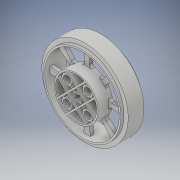
# Autodesk Inventor part: wheel
Saved by Autodesk Inventor 2019 (Build 230136000, 136)
## iProperties
Created: 2019-02-04
Part Number: wheel
Material: Generic
Document SubType Name: Modeling
Designer: david
Density: 1 g/cm^3
Appearance: Default
Author: david
Autodesk Inventor part; units mm, degrees
ref_plane "YZ Plane" through (0, 0, 0) normal (1, 0, 0) x (0, 1, 0)
ref_plane "XZ Plane" through (0, 0, 0) normal (0, 1, 0) x (-1, 0, 0)
ref_plane "XY Plane" through (0, 0, 0) normal (0, 0, 1) x (1, 0, 0)
sketch "Sketch1" plane through (0, 0, 0) normal (0, 0, 1) x (1, 0, 0)
  circle A0 centre (0, 0) radius 15
  dimension "d0" = 30
  constraints: 1 centre point, 1 coincident
  measures "d0" diameter of A0
extrude "Extrusion1" add sketch "Sketch1" along normal blind 10
ref_plane "Work Plane1" through (0, 0, -9) normal (0, 0, -1) x (-1, 0, 0)
sketch "Sketch2" plane through (0, 0, -9) normal (0, 0, -1) x (-1, 0, 0)
  circle A0 centre (0, 0) radius 26.65 construction
  circle A1 centre (0, 0) radius 29.5
  circle A2 centre (0, 0) radius 25.5
  dimension "d4" = 59
  dimension "d5" = 53.3
  dimension "d6" = 51
  constraints: 3 centre point, 3 coincident
  measures "d4" diameter of A1
  measures "d5" diameter of A0
  measures "d6" diameter of A2
extrude "Extrusion2" add sketch "Sketch2" against normal blind 15
sketch "Sketch3" plane through (0, 0, -9) normal (0, 0, -1) x (-1, 0, 0)
  circle A0 centre (0, 0) radius 29.5 projected
  circle A1 centre (0, 0) radius 26.75
  dimension "d9" = 53.5
  constraints: 1 centre point, 1 coincident
  measures "d9" diameter of A1
extrude "Extrusion3" cut sketch "Sketch3" against normal blind 2.1
sketch "Sketch4" plane through (0, 0, 6) normal (0, 0, 1) x (1, 0, 0)
  circle A0 centre (0, 0) radius 29.5 projected
  circle A1 centre (0, 0) radius 26.625
  dimension "d12" = 53.25
  constraints: 1 centre point, 1 coincident
  measures "d12" diameter of A1
extrude "Extrusion4" cut sketch "Sketch4" against normal blind 2.1
sketch "Sketch5" plane through (0, 0, 0) normal (0, 1, 0) x (-1, 0, 0)
  line L0 (15, 10) -> (-15, 10) projected
  line L1 (-25.5, 6) -> (25.5, 6) projected
  line L2 (-15, 0) -> (15, 0) projected
  line L3 (25.5, -9) -> (-25.5, -9) projected
  line L4 (-25.5, 6) -> (-25.5, -9)
  line L5 (-15, 0) -> (-25.5, 0)
  line L6 (-15, 0) -> (-15, 10)
  line L7 (-15, 2.5) -> (-25.5, 2.5)
  line L8 (0, 0) -> (0, 13.089) construction
  dimension "d19" = 2.5
  constraints: 10 end point, 3 point on line, 2 perpendicular, 2 vertical, 1 horizontal
  measures "d19" distance between parallel lines of L5 L7
revolve "Revolution1" add sketch "Sketch5" angle 5 about axis through (0, 0, 0) along (0, 0, 1) and the other way 5 contours L7 L6 L5 L4
pattern_circular "Circular Pattern1" count 8 over 360 about axis through (0, 0, -9) along (0, 0, 1) of "Revolution1"
fillet "Fillet1" radius 2 16 edges at (9.6418, 11.4907, 1.25) (11.4907, 9.6418, 1.25) (14.9429, 1.3073, 1.25) (14.9429, -1.3073, 1.25) (1.3073, 14.9429, 1.25) (-9.6418, 11.4907, 1.25) (-1.3073, 14.9429, 1.25) (-11.4907, 9.6418, 1.25) (-14.9429, -1.3073, 1.25) (-14.9429, 1.3073, 1.25) (-11.4907, -9.6418, 1.25) (-9.6418, -11.4907, 1.25) (9.6418, -11.4907, 1.25) (-1.3073, -14.9429, 1.25) (11.4907, -9.6418, 1.25) (1.3073, -14.9429, 1.25)
sketch "Sketch6" plane through (0, 0, 10) normal (0, 0, 1) x (1, 0, 0)
  circle A0 centre (0, 0) radius 25.5 construction
  line L0 (0, -25.5) -> (0, 25.5)
  circle A1 centre (0, 0) radius 26.625 projected
  line L1 (-25.4984, 25.4984) -> (0, 0)
  line L2 (0, 0) -> (-23.7156, -23.7156)
  circle A2 centre (-7.0711, -7.0711) radius 2.5
  line L3 (0, 0) -> (10.6066, 10.6066)
  circle A3 centre (0, 0) radius 15 construction
  line L4 (0, 0) -> (10.6066, -10.6066)
  circle A4 centre (7.0711, -7.0711) radius 2.5
  circle A5 centre (7.0711, 7.0711) radius 2.5
  circle A6 centre (-7.0711, 7.0711) radius 2.5
  line L5 (1.875, -1.575) -> (1.875, 1.575)
  line L6 (-1.875, 1.575) -> (-1.875, -1.575)
  line L7 (1.575, -1.875) -> (-1.575, -1.875)
  line L8 (1.575, 1.875) -> (-1.575, 1.875)
  circle A7 centre (0, 0) radius 2.5 construction
  arc A8 (1.575, -1.875) -> (1.875, -1.575) centre (1.575, -1.575) ccw
  arc A9 (1.875, 1.575) -> (1.575, 1.875) centre (1.575, 1.575) ccw
  arc A10 (-1.575, 1.875) -> (-1.875, 1.575) centre (-1.575, 1.575) ccw
  arc A11 (-1.875, -1.575) -> (-1.575, -1.875) centre (-1.575, -1.575) ccw
  point P0 (1.875, -1.875)
  point P1 (1.875, 1.875)
  point P2 (-1.875, 1.875)
  point P3 (-1.875, -1.875)
  dimension "d26" = 45
  dimension "d27" = 5
  dimension "d28" = 45
  dimension "d29" = 20
  dimension "d30" = 20
  dimension "d31" = 10
  dimension "d32" = 10
  dimension "d33" = 3.75
  dimension "d34" = 5
  dimension "d35" = 0.3
  constraints: 18 end point, 17 point on line, 12 point on circle, 9 centre point, 8 tangent, 6 equal radius, 2 perpendicular, 2 vertical, 1 coincident, 1 parallel
  measures "d26" angle of L2 L0
  measures "d27" diameter of A2
  measures "d28" angle of L0 L3
  measures "d29" distance of A6.centre A4.centre
  measures "d30" distance of A2.centre A5.centre
  measures "d31" distance of A3.centre A4.centre
  measures "d32" distance of A3.centre A5.centre
  measures "d33" distance of point (1.875, -1.875) point (-1.875, -1.875)
  measures "d34" diameter of A7
  measures "d35" radius of A8
extrude "Extrusion6" cut sketch "Sketch6" against normal through all contours L7 A11 L2 L0 | L0 L4 A8 L7 | L1 A10 L8 L0 | L2 A11 L6 A10 L1 | L0 L8 A9 L3 | L3 A9 L5 A8 L4 | A6 L1 | L1 A6 | A2 L2 | L2 A2 | A5 L3 | L3 A5 | A4 L4 | L4 A4
sketch "Sketch7" plane through (0, 0, 10) normal (0, 0, 1) x (1, 0, 0)
  circle A0 centre (0, 0) radius 14
  line L0 (1.575, -1.875) -> (-1.575, -1.875) construction
  arc A1 (1.575, -1.875) -> (1.875, -1.575) centre (1.575, -1.575) ccw construction
  line L1 (1.875, 1.575) -> (1.875, -1.575) construction
  arc A2 (1.875, 1.575) -> (1.575, 1.875) centre (1.575, 1.575) ccw construction
  line L2 (-1.575, 1.875) -> (1.575, 1.875) construction
  arc A3 (-1.575, 1.875) -> (-1.875, 1.575) centre (-1.575, 1.575) ccw construction
  line L3 (-1.875, -1.575) -> (-1.875, 1.575) construction
  arc A4 (-1.875, -1.575) -> (-1.575, -1.875) centre (-1.575, -1.575) ccw construction
  arc A5 (2.875, 1.575) -> (1.575, 2.875) centre (1.575, 1.575) ccw
  line L4 (2.875, 1.575) -> (2.875, -1.575)
  arc A6 (1.575, -2.875) -> (2.875, -1.575) centre (1.575, -1.575) ccw
  line L5 (1.575, -2.875) -> (-1.575, -2.875)
  arc A7 (-2.875, -1.575) -> (-1.575, -2.875) centre (-1.575, -1.575) ccw
  line L6 (-2.875, -1.575) -> (-2.875, 1.575)
  arc A8 (-1.575, 2.875) -> (-2.875, 1.575) centre (-1.575, 1.575) ccw
  line L7 (-1.575, 2.875) -> (1.575, 2.875)
  circle A9 centre (0, 0) radius 15 construction
  circle A10 centre (7.0711, -7.0711) radius 2.5 construction
  circle A11 centre (-7.0711, -7.0711) radius 2.5 construction
  circle A12 centre (-7.0711, 7.0711) radius 2.5 construction
  circle A13 centre (7.0711, 7.0711) radius 2.5 construction
  circle A14 centre (7.0711, -7.0711) radius 3.5
  circle A15 centre (-7.0711, -7.0711) radius 3.5
  circle A16 centre (-7.0711, 7.0711) radius 3.5
  circle A17 centre (7.0711, 7.0711) radius 3.5
  line L8 (0, 0) -> (-12.3738, -12.3738) construction
  line L9 (0, 0) -> (-12.2798, 12.2798) construction
  line L10 (0, 0) -> (11.8433, 11.8433) construction
  line L11 (0, 0) -> (12.1915, -12.1915) construction
  line L12 (0, 0) -> (0, -14) construction
  line L13 (9.167, -9.8741) -> (9.5396, -10.2467)
  line L14 (9.8741, -9.167) -> (10.2467, -9.5396)
  line L15 (2.875, -2.1679) -> (4.9751, -4.268)
  line L16 (0, -1.4142) -> (0.0105, -1.4037)
  line L17 (-9.5396, 10.2467) -> (-9.167, 9.8741)
  line L18 (-10.2467, 9.5396) -> (-9.8741, 9.167)
  line L19 (-4.9751, 4.268) -> (-2.875, 2.1679)
  line L20 (-4.268, 4.9751) -> (-2.1679, 2.875)
  line L21 (4.268, 4.9751) -> (2.1679, 2.875)
  line L22 (4.9751, 4.268) -> (2.875, 2.1679)
  line L23 (-4.9751, -4.268) -> (-2.875, -2.1679)
  line L24 (-4.268, -4.9751) -> (-2.1679, -2.875)
  line L25 (-9.5396, -10.2467) -> (-9.167, -9.8741)
  line L26 (-10.2467, -9.5396) -> (-9.8741, -9.167)
  line L27 (9.5396, 10.2467) -> (9.167, 9.8741)
  line L28 (10.2467, 9.5396) -> (9.8741, 9.167)
  line L29 (2.1679, -2.875) -> (4.268, -4.9751)
  line L30 (2.1679, -2.875) -> (2.07, -2.7771)
  line L31 (2.875, -2.1679) -> (2.7771, -2.07)
  line L32 (-2.1679, -2.875) -> (-2.07, -2.7771)
  line L33 (-2.875, -2.1679) -> (-2.7771, -2.07)
  line L34 (-2.1679, 2.875) -> (-2.07, 2.7771)
  line L35 (-2.875, 2.1679) -> (-2.7771, 2.07)
  line L36 (2.1679, 2.875) -> (2.07, 2.7771)
  line L37 (2.875, 2.1679) -> (2.7771, 2.07)
  dimension "d40" = 1
  dimension "d41" = 1
  dimension "d42" = 1
  dimension "d43" = 45
  dimension "d52" = 0.5
  dimension "d53" = 0.5
  dimension "d54" = 0.5
  dimension "d55" = 0.5
  constraints: 68 end point, 32 point on circle, 14 collinear, 13 perpendicular, 8 centre point, 8 point on line, 4 parallel, 3 equal radius, 1 coincident, 1 vertical, 18 other
  measures "d40" distance between parallel lines of L6 L3
  measures "d42" radial gap between concentric circles of A14 A10
  measures "d43" angle of L8 L12
  measures "d52" distance between parallel lines of L29 L11
  measures "d53" distance between parallel lines of L15 L11
  measures "d54" distance between parallel lines of L23 L8
  measures "d55" distance between parallel lines of L8 L24
extrude "Extrusion9" cut sketch "Sketch7" against normal blind 4.5 contours A0 L14 A14 L15 L31 A6 L4 A5 L37 L22 A17 L28 | L27 A17 L21 L36 A5 L7 A8 L34 L20 A16 L17 A0 | A0 L25 A15 L24 L32 A7 L5 A6 L30 L29 A14 L13 | L18 A16 L19 L35 A8 L6 A7 L33 L23 A15 L26 A0
sketch "Sketch8" plane through (0, 0, 0) normal (0, 0, -1) x (-1, 0, 0)
  arc A0 (-9.167, -9.8741) -> (-4.268, -4.9751) centre (-7.0711, -7.0711) ccw projected
  line L0 (-2.07, -2.7771) -> (-4.268, -4.9751) projected
  line L1 (-9.167, -9.8741) -> (-9.5396, -10.2467) projected
  arc A1 (-9.5396, -10.2467) -> (9.5396, -10.2467) centre (0, 0) ccw projected
  arc A2 (-10.2467, 9.5396) -> (-10.2467, -9.5396) centre (0, 0) ccw projected
  line L2 (-10.2467, -9.5396) -> (-9.8741, -9.167) projected
  arc A3 (-4.9751, -4.268) -> (-9.8741, -9.167) centre (-7.0711, -7.0711) ccw projected
  line L3 (-4.9751, -4.268) -> (-2.7771, -2.07) projected
  line L4 (1.575, -2.875) -> (-1.575, -2.875) projected
  line L5 (-2.875, -1.575) -> (-2.875, 1.575) projected
  arc A4 (-2.875, -1.575) -> (-2.7771, -2.07) centre (-1.575, -1.575) ccw projected
  arc A5 (-2.07, -2.7771) -> (-1.575, -2.875) centre (-1.575, -1.575) ccw projected
  line L6 (-1.575, 2.875) -> (1.575, 2.875) projected
  line L7 (2.7771, -2.07) -> (4.9751, -4.268) projected
  line L8 (4.268, -4.9751) -> (2.07, -2.7771) projected
  arc A6 (4.268, -4.9751) -> (9.167, -9.8741) centre (7.0711, -7.0711) ccw projected
  arc A7 (9.8741, -9.167) -> (4.9751, -4.268) centre (7.0711, -7.0711) ccw projected
  line L9 (9.8741, -9.167) -> (10.2467, -9.5396) projected
  line L10 (9.5396, -10.2467) -> (9.167, -9.8741) projected
  arc A8 (10.2467, -9.5396) -> (10.2467, 9.5396) centre (0, 0) ccw projected
  arc A9 (9.5396, 10.2467) -> (-9.5396, 10.2467) centre (0, 0) ccw projected
  line L11 (4.9751, 4.268) -> (2.7771, 2.07) projected
  line L12 (2.07, 2.7771) -> (4.268, 4.9751) projected
  arc A10 (9.167, 9.8741) -> (4.268, 4.9751) centre (7.0711, 7.0711) ccw projected
  arc A11 (4.9751, 4.268) -> (9.8741, 9.167) centre (7.0711, 7.0711) ccw projected
  line L13 (10.2467, 9.5396) -> (9.8741, 9.167) projected
  line L14 (9.167, 9.8741) -> (9.5396, 10.2467) projected
  line L15 (-4.268, 4.9751) -> (-2.07, 2.7771) projected
  line L16 (-2.7771, 2.07) -> (-4.9751, 4.268) projected
  arc A12 (-9.8741, 9.167) -> (-4.9751, 4.268) centre (-7.0711, 7.0711) ccw projected
  arc A13 (-4.268, 4.9751) -> (-9.167, 9.8741) centre (-7.0711, 7.0711) ccw projected
  line L17 (-9.5396, 10.2467) -> (-9.167, 9.8741) projected
  line L18 (-9.8741, 9.167) -> (-10.2467, 9.5396) projected
  line L19 (2.875, 1.575) -> (2.875, -1.575) projected
  arc A14 (2.875, 1.575) -> (2.7771, 2.07) centre (1.575, 1.575) ccw projected
  arc A15 (2.07, 2.7771) -> (1.575, 2.875) centre (1.575, 1.575) ccw projected
  arc A16 (-1.575, 2.875) -> (-2.07, 2.7771) centre (-1.575, 1.575) ccw projected
  arc A17 (-2.7771, 2.07) -> (-2.875, 1.575) centre (-1.575, 1.575) ccw projected
  arc A18 (1.575, -2.875) -> (2.07, -2.7771) centre (1.575, -1.575) ccw projected
  arc A19 (2.7771, -2.07) -> (2.875, -1.575) centre (1.575, -1.575) ccw projected
extrude "Extrusion10" cut sketch "Sketch8" against normal blind 4.5
sketch "Sketch9" plane through (0, 0, 10) normal (0, 0, 1) x (1, 0, 0)
  arc A0 (-9.5396, -10.2467) -> (9.5396, -10.2467) centre (0, 0) ccw projected
  circle A1 centre (0, 0) radius 14
  constraints: 1 coincident, 3 other
extrude "Extrusion11" cut sketch "Sketch9" against normal blind 0.8
sketch "Sketch10" plane through (0, 0, 0) normal (0, 0, -1) x (-1, 0, 0)
  line L0 (-9.5396, -10.2467) -> (-9.167, -9.8741) projected
  circle A0 centre (0, 0) radius 14
  constraints: 1 coincident, 3 other
extrude "Extrusion12" cut sketch "Sketch10" against normal blind 0.8
sketch "Sketch12" plane through (0, 0, 5.5) normal (0, 0, 1) x (1, 0, 0)
  circle A0 centre (-7.0711, -7.0711) radius 2.5 projected
  circle A1 centre (7.0711, 7.0711) radius 2.5 projected
  line L0 (-7.0711, -7.0711) -> (7.0711, 7.0711) construction
  line L1 (-12.7822, -5.7111) -> (5.7111, 12.7822)
  line L2 (-5.7111, -12.7822) -> (12.7822, 5.7111)
  circle A2 centre (0, 0) radius 14 projected
  line L3 (-12.3153, -6.6584) -> (6.6584, 12.3153)
  line L4 (-6.6584, -12.3153) -> (12.3153, 6.6584)
  circle A3 centre (-7.0711, 7.0711) radius 2.5 projected
  circle A4 centre (7.0711, -7.0711) radius 2.5 projected
  line L5 (-7.0711, 7.0711) -> (7.0711, -7.0711) construction
  line L6 (-6.6584, 12.3153) -> (12.3153, -6.6584)
  line L7 (-5.7111, 12.7822) -> (12.7822, -5.7111)
  line L8 (-12.7822, 5.7111) -> (5.7111, -12.7822)
  line L9 (-12.3153, 6.6584) -> (6.6584, -12.3153)
  dimension "d72" = 5
  dimension "d73" = 5
  dimension "d74" = 1
  dimension "d75" = 1
  dimension "d76" = 5
  dimension "d77" = 1
  dimension "d78" = 4
  dimension "d79" = 1
  constraints: 20 end point, 8 parallel, 17 other
  measures "d72" distance between parallel lines of L0 L1
  measures "d73" distance between parallel lines of L2 L0
  measures "d74" distance between parallel lines of L1 L3
  measures "d75" distance between parallel lines of L2 L4
  measures "d76" distance between parallel lines of L5 L7
  measures "d77" distance between parallel lines of L7 L6
  measures "d78" distance between parallel lines of L5 L9
  measures "d79" distance between parallel lines of L8 L9
extrude "Extrusion14" add sketch "Sketch12" along normal up to surface (4.5 mm away) contours L1 L8 L3 A2 | L8 A2 L9 L1 | L1 L9 L3 L8 | L1 L6 L3 L9 | L3 L9 L4 L8 | L4 L8 L2 A2 | L6 A2 L7 L1 | L1 L7 L3 L6 | L4 L9 L2 L8 | L1 A2 L3 L7 | L3 L7 L4 L6 | L4 L6 L2 L9 | L2 L9 A2 L8 | L4 L7 L2 L6 | L4 A2 L2 L7 | L2 L7 A2 L6
sketch "Sketch13" plane through (0, 0, 5.5) normal (0, 0, 1) x (1, 0, 0)
  circle A0 centre (7.0711, -7.0711) radius 2.5 construction
  line L0 (7.0711, -7.0711) -> (9.8995, -4.2426) construction
  line L1 (12.3153, -6.6584) -> (6.364, -0.7071) construction
  line L2 (7.0596, -7.0826) -> (11.3798, -7.0826) construction
  arc A1 (4.268, -4.9751) -> (9.167, -9.8741) centre (7.0711, -7.0711) ccw construction
  arc A2 (9.8741, -9.167) -> (4.9751, -4.268) centre (7.0711, -7.0711) ccw construction
  arc A3 (-9.8741, 9.167) -> (-4.9751, 4.268) centre (-7.0711, 7.0711) ccw construction
  arc A4 (-4.268, 4.9751) -> (-9.167, 9.8741) centre (-7.0711, 7.0711) ccw construction
  line L3 (-7.0711, 7.0711) -> (-5.3143, 8.8279) construction
  line L4 (-0.7071, 6.364) -> (-6.6584, 12.3153) construction
  line L5 (2.4749, 3.182) -> (0, 5.6569) construction
  line L6 (6.6584, 12.3153) -> (0.7071, 6.364) construction
  line L7 (0, 7.0711) -> (5.7111, 12.7822) construction
  line L8 (-5.7111, 12.7822) -> (0, 7.0711) construction
  line L9 (-12.3153, 6.6584) -> (-6.364, 0.7071) projected
  line L10 (-6.364, -0.7071) -> (-12.3153, -6.6584) construction
  line L11 (-6.6584, -12.3153) -> (-0.7071, -6.364) construction
  line L12 (0.7071, -6.364) -> (6.6584, -12.3153) construction
  line L13 (-10.253, 4.5962) -> (-9.8741, 4.9751)
  line L14 (-4.9751, 9.8741) -> (-4.5962, 10.253)
  line L15 (-9.5459, 3.8891) -> (-9.167, 4.268)
  line L16 (-4.268, 9.167) -> (-3.8891, 9.5459)
  line L17 (3.8814, -9.5536) -> (4.268, -9.167)
  line L18 (9.167, -4.268) -> (9.5459, -3.8891)
  line L19 (9.8741, -4.9751) -> (10.253, -4.5962)
  line L20 (4.5886, -10.2607) -> (4.9751, -9.8741)
  circle A5 centre (-7.0711, -7.0711) radius 2.5 construction
  line L21 (-7.0711, -7.0711) -> (-8.8388, -5.3033) construction
  line L22 (-7.0711, -7.0711) -> (-9.5711, -7.0711) construction
  arc A6 (-9.167, -9.8741) -> (-4.268, -4.9751) centre (-7.0711, -7.0711) ccw construction
  arc A7 (-4.9751, -4.268) -> (-9.8741, -9.167) centre (-7.0711, -7.0711) ccw construction
  line L23 (-9.5459, -3.8891) -> (-9.167, -4.268)
  line L24 (-4.268, -9.167) -> (-3.8891, -9.5459)
  line L25 (-10.253, -4.5962) -> (-9.8741, -4.9751)
  line L26 (-4.9751, -9.8741) -> (-4.5962, -10.253)
  circle A8 centre (7.0711, 7.0711) radius 2.5 construction
  line L27 (7.0711, 7.0711) -> (4.2426, 9.8995) construction
  line L28 (6.6584, 12.3153) -> (0.7071, 6.364) construction
  line L29 (7.0711, 7.0711) -> (9.5711, 7.0711) construction
  line L30 (6.364, 0.7071) -> (12.3153, 6.6584) construction
  arc A9 (4.9751, 4.268) -> (9.8741, 9.167) centre (7.0711, 7.0711) ccw construction
  arc A10 (9.167, 9.8741) -> (4.268, 4.9751) centre (7.0711, 7.0711) ccw construction
  line L31 (10.3232, 4.526) -> (9.8741, 4.9751)
  line L32 (4.9751, 9.8741) -> (4.5962, 10.253)
  line L33 (9.6161, 3.8189) -> (9.167, 4.268)
  line L34 (4.268, 9.167) -> (3.8891, 9.5459)
  line L35 (-4.268, 4.9751) -> (-3.182, 3.8891) construction
  arc A11 (-4.268, 4.9751) -> (-9.167, 9.8741) centre (-7.0711, 7.0711) ccw construction
  line L36 (-9.5396, 10.2467) -> (-9.167, 9.8741) construction
  arc A12 (-9.5396, 10.2467) -> (-10.2467, 9.5396) centre (0, 0) ccw construction
  line L37 (-9.8741, 9.167) -> (-10.2467, 9.5396) construction
  arc A13 (-9.8741, 9.167) -> (-4.9751, 4.268) centre (-7.0711, 7.0711) ccw projected
  line L38 (-3.8891, 3.182) -> (-4.9751, 4.268) construction
  line L39 (-4.9751, -4.268) -> (-3.8891, -3.182) construction
  arc A14 (-4.9751, -4.268) -> (-9.8741, -9.167) centre (-7.0711, -7.0711) ccw construction
  line L40 (-10.2467, -9.5396) -> (-9.8741, -9.167) construction
  arc A15 (-10.2467, -9.5396) -> (-9.5396, -10.2467) centre (0, 0) ccw construction
  line L41 (-9.167, -9.8741) -> (-9.5396, -10.2467) construction
  arc A16 (-9.167, -9.8741) -> (-4.268, -4.9751) centre (-7.0711, -7.0711) ccw construction
  line L42 (-3.182, -3.8891) -> (-4.268, -4.9751) construction
  line L43 (4.268, -4.9751) -> (3.182, -3.8891) construction
  arc A17 (4.268, -4.9751) -> (9.167, -9.8741) centre (7.0711, -7.0711) ccw construction
  line L44 (9.5396, -10.2467) -> (9.167, -9.8741) construction
  arc A18 (9.5396, -10.2467) -> (10.2467, -9.5396) centre (0, 0) ccw construction
  line L45 (9.8741, -9.167) -> (10.2467, -9.5396) construction
  arc A19 (9.8741, -9.167) -> (4.9751, -4.268) centre (7.0711, -7.0711) ccw construction
  line L46 (3.8891, -3.182) -> (4.9751, -4.268) construction
  line L47 (4.9751, 4.268) -> (3.8891, 3.182) construction
  arc A20 (4.9751, 4.268) -> (9.8741, 9.167) centre (7.0711, 7.0711) ccw construction
  line L48 (10.2467, 9.5396) -> (9.8741, 9.167) construction
  arc A21 (10.2467, 9.5396) -> (9.5396, 10.2467) centre (0, 0) ccw construction
  line L49 (9.167, 9.8741) -> (9.5396, 10.2467) construction
  arc A22 (9.167, 9.8741) -> (4.268, 4.9751) centre (7.0711, 7.0711) ccw construction
  line L50 (3.182, 3.8891) -> (4.268, 4.9751) construction
  line L51 (-2.7771, 2.07) -> (-3.182, 2.4749) construction
  arc A23 (-2.7771, 2.07) -> (-2.875, 1.575) centre (-1.575, 1.575) ccw construction
  line L52 (-2.875, -1.575) -> (-2.875, 1.575) construction
  arc A24 (-2.875, -1.575) -> (-2.7771, -2.07) centre (-1.575, -1.575) ccw construction
  line L53 (-3.182, -2.4749) -> (-2.7771, -2.07) construction
  line L54 (2.07, 2.7771) -> (2.4749, 3.182) construction
  arc A25 (2.07, 2.7771) -> (1.575, 2.875) centre (1.575, 1.575) ccw construction
  line L55 (-1.575, 2.875) -> (1.575, 2.875) construction
  arc A26 (-1.575, 2.875) -> (-2.07, 2.7771) centre (-1.575, 1.575) ccw construction
  line L56 (-2.4749, 3.182) -> (-2.07, 2.7771) construction
  line L57 (-2.07, -2.7771) -> (-2.4749, -3.182) construction
  arc A27 (-2.07, -2.7771) -> (-1.575, -2.875) centre (-1.575, -1.575) ccw construction
  line L58 (1.575, -2.875) -> (-1.575, -2.875) construction
  arc A28 (1.575, -2.875) -> (2.07, -2.7771) centre (1.575, -1.575) ccw construction
  line L59 (2.4749, -3.182) -> (2.07, -2.7771) construction
  circle A29 centre (7.0711, 7.0711) radius 2.5 construction
  circle A30 centre (-7.0711, -7.0711) radius 2.5 construction
  circle A31 centre (7.0711, -7.0711) radius 2.5 construction
  arc A32 (-1.875, -1.575) -> (-1.575, -1.875) centre (-1.575, -1.575) ccw construction
  line L60 (-1.875, 1.575) -> (-1.875, -1.575) construction
  arc A33 (-1.575, 1.875) -> (-1.875, 1.575) centre (-1.575, 1.575) ccw construction
  line L61 (1.575, 1.875) -> (-1.575, 1.875) construction
  arc A34 (1.875, 1.575) -> (1.575, 1.875) centre (1.575, 1.575) ccw construction
  line L62 (1.875, -1.575) -> (1.875, 1.575) construction
  arc A35 (1.575, -1.875) -> (1.875, -1.575) centre (1.575, -1.575) ccw construction
  line L63 (-1.575, -1.875) -> (1.575, -1.875) construction
  line L64 (2.7771, -2.07) -> (3.182, -2.4749) construction
  arc A36 (2.7771, -2.07) -> (2.875, -1.575) centre (1.575, -1.575) ccw construction
  line L65 (2.875, 1.575) -> (2.875, -1.575) construction
  arc A37 (2.875, 1.575) -> (2.7771, 2.07) centre (1.575, 1.575) ccw construction
  line L66 (3.182, 2.4749) -> (2.7771, 2.07) construction
  circle A38 centre (-7.0711, 7.0711) radius 2.5 construction
  line L67 (-10.253, 4.5962) -> (-9.5459, 3.8891)
  line L68 (-12.3153, 6.6584) -> (-6.364, 0.7071) projected
  arc A39 (-9.8741, 4.9751) -> (-9.167, 4.268) centre (-7.0711, 7.0711) ccw
  line L69 (-10.253, -4.5962) -> (-9.5459, -3.8891)
  line L70 (-6.364, -0.7071) -> (-12.3153, -6.6584) projected
  line L71 (-4.5962, -10.253) -> (-3.8891, -9.5459)
  line L72 (10.253, -4.5962) -> (9.5459, -3.8891)
  line L73 (9.6161, 3.8189) -> (10.3232, 4.526)
  line L74 (6.364, 0.7071) -> (12.3153, 6.6584) projected
  line L75 (-4.5962, 10.253) -> (-3.8891, 9.5459)
  line L76 (3.8891, 9.5459) -> (4.5962, 10.253)
  arc A40 (-4.268, 9.167) -> (-4.9751, 9.8741) centre (-7.0711, 7.0711) ccw
  arc A41 (4.9751, 9.8741) -> (4.268, 9.167) centre (7.0711, 7.0711) ccw
  arc A42 (9.167, 4.268) -> (9.8741, 4.9751) centre (7.0711, 7.0711) ccw
  arc A43 (-4.9751, -9.8741) -> (-4.268, -9.167) centre (-7.0711, -7.0711) ccw
  arc A44 (9.8741, -4.9751) -> (9.167, -4.268) centre (7.0711, -7.0711) ccw
  arc A45 (-9.167, -4.268) -> (-9.8741, -4.9751) centre (-7.0711, -7.0711) ccw
  line L77 (3.8814, -9.5536) -> (4.5886, -10.2607)
  line L78 (0.7071, -6.364) -> (6.6584, -12.3153) projected
  arc A46 (4.268, -9.167) -> (4.9751, -9.8741) centre (7.0711, -7.0711) ccw
  line L79 (-3.182, -3.8891) -> (-3.8891, -3.182) projected
  line L80 (-3.182, -2.4749) -> (-2.4749, -3.182) projected
  line L81 (2.4749, -3.182) -> (3.182, -2.4749) projected
  line L82 (3.182, 2.4749) -> (2.4749, 3.182) projected
  line L83 (-2.4749, 3.182) -> (-3.182, 2.4749) projected
  line L84 (3.182, 3.8891) -> (3.8891, 3.182) projected
  line L85 (-3.8891, 3.182) -> (-3.182, 3.8891) projected
  line L86 (3.8891, -3.182) -> (3.182, -3.8891) projected
  point P0 (-6.364, 0.7071)
  point P1 (-6.364, -0.7071)
  point P2 (0.7071, -6.364)
  point P3 (6.364, 0.7071)
  dimension "d82" = 45
  dimension "d87" = 45
  dimension "d90" = 45
  dimension "d93" = 0.5
  dimension "d95" = 0.5
  constraints: 62 end point, 34 point on circle, 20 parallel, 8 centre point, 7 point on line, 4 concentric, 3 horizontal, 2 collinear, 2 perpendicular, 1 horizontal alignment, 3 other
  measures "d82" angle of L2 L0
  measures "d87" angle of L22 L21
  measures "d90" angle of L29 L27
  measures "d93" distance between parallel lines of L3 L13
  measures "d95" distance between parallel lines of L3 L15
extrude "Extrusion15" add sketch "Sketch13" along normal up to surface (3.7 mm away)
sketch "Sketch14" plane through (0, 0, 4.5) normal (0, 0, -1) x (-1, 0, 0)
  arc A0 (9.8741, -9.167) -> (4.9751, -4.268) centre (7.0711, -7.0711) ccw projected
  arc A1 (-9.167, -9.8741) -> (-4.9751, -9.8741) centre (-7.0711, -7.0711) ccw projected
  line L0 (-9.5396, -10.2467) -> (-9.167, -9.8741) projected
  arc A2 (-10.2467, -9.5396) -> (-9.5396, -10.2467) centre (0, 0) ccw projected
  line L1 (-9.8741, -9.167) -> (-10.2467, -9.5396) projected
  arc A3 (-9.8741, -4.9751) -> (-9.8741, -9.167) centre (-7.0711, -7.0711) ccw projected
  line L2 (-10.253, -4.5962) -> (-9.8741, -4.9751) projected
  line L3 (-9.8741, 4.9751) -> (-10.253, 4.5962) projected
  arc A4 (-9.8741, 9.167) -> (-9.8741, 4.9751) centre (-7.0711, 7.0711) ccw projected
  line L4 (-10.2467, 9.5396) -> (-9.8741, 9.167) projected
  arc A5 (-9.5396, 10.2467) -> (-10.2467, 9.5396) centre (0, 0) ccw projected
  line L5 (-9.167, 9.8741) -> (-9.5396, 10.2467) projected
  arc A6 (-4.9751, 9.8741) -> (-9.167, 9.8741) centre (-7.0711, 7.0711) ccw projected
  line L6 (-4.5962, 10.253) -> (-4.9751, 9.8741) projected
  line L7 (4.9751, 9.8741) -> (4.5962, 10.253) projected
  arc A7 (9.167, 9.8741) -> (4.9751, 9.8741) centre (7.0711, 7.0711) ccw projected
  line L8 (9.5396, 10.2467) -> (9.167, 9.8741) projected
  arc A8 (10.2467, 9.5396) -> (9.5396, 10.2467) centre (0, 0) ccw projected
  line L9 (9.8741, 9.167) -> (10.2467, 9.5396) projected
  arc A9 (9.8741, 4.9751) -> (9.8741, 9.167) centre (7.0711, 7.0711) ccw projected
  line L10 (10.253, 4.5962) -> (9.8741, 4.9751) projected
  line L11 (9.8741, -4.9751) -> (10.253, -4.5962) projected
  arc A10 (9.8741, -9.167) -> (9.8741, -4.9751) centre (7.0711, -7.0711) ccw projected
  line L12 (10.2467, -9.5396) -> (9.8741, -9.167) projected
  arc A11 (9.5396, -10.2467) -> (10.2467, -9.5396) centre (0, 0) ccw projected
  line L13 (9.167, -9.8741) -> (9.5396, -10.2467) projected
  arc A12 (4.9751, -9.8741) -> (9.167, -9.8741) centre (7.0711, -7.0711) ccw projected
  line L14 (4.5962, -10.253) -> (4.9751, -9.8741) projected
  line L15 (-4.9751, -9.8741) -> (-4.5962, -10.253) projected
  line L16 (-4.9751, 4.268) -> (-3.8891, 3.182) projected
  arc A13 (-9.167, 4.268) -> (-4.9751, 4.268) centre (-7.0711, 7.0711) ccw projected
  line L17 (-9.5459, 3.8891) -> (-9.167, 4.268) projected
  arc A14 (-4.268, 4.9751) -> (-4.268, 9.167) centre (-7.0711, 7.0711) ccw projected
  line L18 (-3.182, 3.8891) -> (-4.268, 4.9751) projected
  line L19 (-4.268, 9.167) -> (-3.8891, 9.5459) projected
  line L20 (4.9751, -4.268) -> (3.8891, -3.182) projected
  arc A15 (9.167, -4.268) -> (4.9751, -4.268) centre (7.0711, -7.0711) ccw projected
  line L21 (9.5459, -3.8891) -> (9.167, -4.268) projected
  arc A16 (4.9751, 4.268) -> (9.167, 4.268) centre (7.0711, 7.0711) ccw projected
  line L22 (3.8891, 3.182) -> (4.9751, 4.268) projected
  line L23 (9.167, 4.268) -> (9.5459, 3.8891) projected
  line L24 (-3.8891, -9.5459) -> (-4.268, -9.167) projected
  line L25 (-4.268, -4.9751) -> (-3.182, -3.8891) projected
  arc A17 (-4.268, -9.167) -> (-4.268, -4.9751) centre (-7.0711, -7.0711) ccw projected
  line L26 (-9.167, -4.268) -> (-9.5459, -3.8891) projected
  arc A18 (-4.9751, -4.268) -> (-9.167, -4.268) centre (-7.0711, -7.0711) ccw projected
  line L27 (-3.8891, -3.182) -> (-4.9751, -4.268) projected
  line L28 (3.8891, 9.5459) -> (4.268, 9.167) projected
  line L29 (4.268, 4.9751) -> (3.182, 3.8891) projected
  arc A19 (4.268, 9.167) -> (4.268, 4.9751) centre (7.0711, 7.0711) ccw projected
  line L30 (4.268, -9.167) -> (3.8891, -9.5459) projected
  arc A20 (4.268, -4.9751) -> (4.268, -9.167) centre (7.0711, -7.0711) ccw projected
  line L31 (3.182, -3.8891) -> (4.268, -4.9751) projected
  line L32 (2.7771, 2.07) -> (3.182, 2.4749) projected
  arc A21 (2.875, 1.575) -> (2.7771, 2.07) centre (1.575, 1.575) ccw projected
  line L33 (2.875, -1.575) -> (2.875, 1.575) projected
  arc A22 (2.7771, -2.07) -> (2.875, -1.575) centre (1.575, -1.575) ccw projected
  line L34 (3.182, -2.4749) -> (2.7771, -2.07) projected
  line L35 (-2.07, 2.7771) -> (-2.4749, 3.182) projected
  arc A23 (-1.575, 2.875) -> (-2.07, 2.7771) centre (-1.575, 1.575) ccw projected
  line L36 (1.575, 2.875) -> (-1.575, 2.875) projected
  arc A24 (2.07, 2.7771) -> (1.575, 2.875) centre (1.575, 1.575) ccw projected
  line L37 (2.4749, 3.182) -> (2.07, 2.7771) projected
  line L38 (2.07, -2.7771) -> (2.4749, -3.182) projected
  arc A25 (1.575, -2.875) -> (2.07, -2.7771) centre (1.575, -1.575) ccw projected
  line L39 (-1.575, -2.875) -> (1.575, -2.875) projected
  arc A26 (-2.07, -2.7771) -> (-1.575, -2.875) centre (-1.575, -1.575) ccw projected
  line L40 (-2.4749, -3.182) -> (-2.07, -2.7771) projected
  circle A27 centre (-7.0711, 7.0711) radius 2.5 projected
  circle A28 centre (7.0711, -7.0711) radius 2.5 projected
  circle A29 centre (-7.0711, -7.0711) radius 2.5 projected
  arc A30 (1.575, -1.875) -> (1.875, -1.575) centre (1.575, -1.575) ccw projected
  line L41 (1.875, 1.575) -> (1.875, -1.575) projected
  arc A31 (1.875, 1.575) -> (1.575, 1.875) centre (1.575, 1.575) ccw projected
  line L42 (-1.575, 1.875) -> (1.575, 1.875) projected
  arc A32 (-1.575, 1.875) -> (-1.875, 1.575) centre (-1.575, 1.575) ccw projected
  line L43 (-1.875, -1.575) -> (-1.875, 1.575) projected
  arc A33 (-1.875, -1.575) -> (-1.575, -1.875) centre (-1.575, -1.575) ccw projected
  line L44 (1.575, -1.875) -> (-1.575, -1.875) projected
  line L45 (-2.7771, -2.07) -> (-3.182, -2.4749) projected
  arc A34 (-2.875, -1.575) -> (-2.7771, -2.07) centre (-1.575, -1.575) ccw projected
  line L46 (-2.875, 1.575) -> (-2.875, -1.575) projected
  arc A35 (-2.7771, 2.07) -> (-2.875, 1.575) centre (-1.575, 1.575) ccw projected
  line L47 (-3.182, 2.4749) -> (-2.7771, 2.07) projected
  circle A36 centre (7.0711, 7.0711) radius 2.5 projected
  line L48 (3.182, -3.8891) -> (3.8891, -3.182) projected
  line L49 (10.253, -4.5962) -> (9.5459, -3.8891) projected
  line L50 (3.8891, -9.5459) -> (4.5962, -10.253) projected
  line L51 (3.182, -2.4749) -> (2.4749, -3.182) projected
  line L52 (-2.4749, -3.182) -> (-3.182, -2.4749) projected
  line L53 (-3.182, 2.4749) -> (-2.4749, 3.182) projected
  line L54 (2.4749, 3.182) -> (3.182, 2.4749) projected
  line L55 (-3.182, 3.8891) -> (-3.8891, 3.182) projected
  line L56 (-10.253, 4.5962) -> (-9.5459, 3.8891) projected
  line L57 (-3.8891, 9.5459) -> (-4.5962, 10.253) projected
  line L58 (3.8891, 3.182) -> (3.182, 3.8891) projected
  line L59 (4.5962, 10.253) -> (3.8891, 9.5459) projected
  line L60 (9.5459, 3.8891) -> (10.253, 4.5962) projected
  line L61 (-3.8891, -3.182) -> (-3.182, -3.8891) projected
  line L62 (-4.5962, -10.253) -> (-3.8891, -9.5459) projected
  line L63 (-9.5459, -3.8891) -> (-10.253, -4.5962) projected
  point P0 (6.364, 0.7071)
sketch "Sketch15" plane through (0, 0, 4.5) normal (0, 0, -1) x (-1, 0, 0)
  arc A0 (6.6584, -12.3153) -> (12.3153, -6.6584) centre (0, 0) ccw projected
  line L0 (6.364, -0.7071) -> (12.3153, -6.6584) projected
  line L1 (0.7071, -6.364) -> (6.364, -0.7071) projected
  line L2 (6.6584, -12.3153) -> (0.7071, -6.364) projected
  line L3 (0, -7.0711) -> (5.7111, -12.7822) projected
  line L4 (-5.7111, -12.7822) -> (0, -7.0711) projected
  arc A1 (-5.7111, -12.7822) -> (5.7111, -12.7822) centre (0, 0) ccw projected
  arc A2 (12.7822, -5.7111) -> (12.7822, 5.7111) centre (0, 0) ccw projected
  line L5 (7.0711, 0) -> (12.7822, 5.7111) projected
  line L6 (12.7822, -5.7111) -> (7.0711, 0) projected
  arc A3 (12.3153, 6.6584) -> (6.6584, 12.3153) centre (0, 0) ccw projected
  line L7 (0.7071, 6.364) -> (6.6584, 12.3153) projected
  line L8 (6.364, 0.7071) -> (0.7071, 6.364) projected
  line L9 (12.3153, 6.6584) -> (6.364, 0.7071) projected
  line L10 (-0.7071, -6.364) -> (-6.6584, -12.3153) projected
  line L11 (-6.364, -0.7071) -> (-0.7071, -6.364) projected
  line L12 (-12.3153, -6.6584) -> (-6.364, -0.7071) projected
  arc A4 (-12.3153, -6.6584) -> (-6.6584, -12.3153) centre (0, 0) ccw projected
  line L13 (-7.0711, 0) -> (-12.7822, -5.7111) projected
  line L14 (-12.7822, 5.7111) -> (-7.0711, 0) projected
  arc A5 (-12.7822, 5.7111) -> (-12.7822, -5.7111) centre (0, 0) ccw projected
  arc A6 (5.7111, 12.7822) -> (-5.7111, 12.7822) centre (0, 0) ccw projected
  line L15 (0, 7.0711) -> (-5.7111, 12.7822) projected
  line L16 (5.7111, 12.7822) -> (0, 7.0711) projected
  line L17 (5.6569, 0) -> (0, -5.6569) projected
  line L18 (0, 5.6569) -> (5.6569, 0) projected
  line L19 (-5.6569, 0) -> (0, 5.6569) projected
  line L20 (0, -5.6569) -> (-5.6569, 0) projected
  circle A7 centre (0, 0) radius 15 projected
  line L21 (-6.364, 0.7071) -> (-12.3153, 6.6584) projected
  line L22 (-0.7071, 6.364) -> (-6.364, 0.7071) projected
  line L23 (-6.6584, 12.3153) -> (-0.7071, 6.364) projected
  arc A8 (-6.6584, 12.3153) -> (-12.3153, 6.6584) centre (0, 0) ccw projected
extrude "Extrusion17" add sketch "Sketch15" along normal up to surface (4.5 mm away)
extrude "Extrusion18" add sketch "Sketch14" along normal up to surface (3.7 mm away) contours L12 A11 L13 A12 L14 L50 L30 A20 L31 L48 L20 A0 | A0 L21 L49 L11 | L0 A2 L1 A3 L2 L63 L26 A18 L27 L61 L25 A17 L24 L62 L15 A1 | A4 L4 A5 L5 A6 L6 L57 L19 A14 L18 L55 L16 A13 L17 L56 L3 | A7 L8 A8 L9 A9 L10 L60 L23 A16 L22 L58 L29 A19 L28 L59 L7
body "Solid1"
